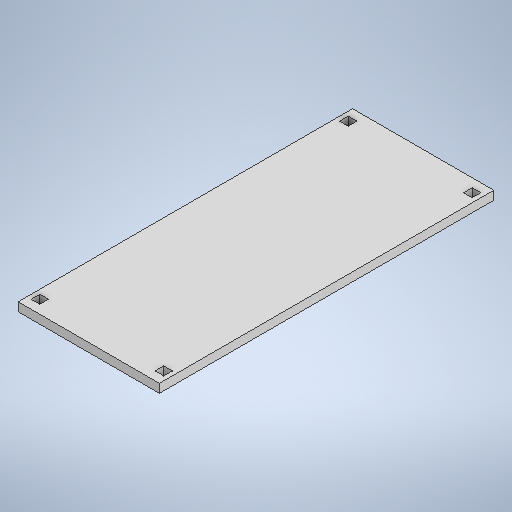
# Autodesk Inventor part: Platform_Arm_2
Saved by Autodesk Inventor 2025 (Build 290162000, 162)
## iProperties
Created: 2024-06-25
Part Number: Platform_Arm_2
Material: Generic
Document SubType Name: Modeling
Designer: User
Density: 1 g/cm^3
Appearance: Default
Author: User
Autodesk Inventor part; units mm, degrees
ref_plane "YZ Plane" through (0, 0, 0) normal (1, 0, 0) x (0, 1, 0)
ref_plane "XZ Plane" through (0, 0, 0) normal (0, 1, 0) x (-1, 0, 0)
ref_plane "XY Plane" through (0, 0, 0) normal (0, 0, 1) x (1, 0, 0)
sketch "Sketch1" plane through (0, 0, 0) normal (0, 1, 0) x (-1, 0, 0)
  line L0 (-245, 580) -> (245, 580)
  line L1 (245, 580) -> (245, -580)
  line L2 (245, -580) -> (-245, -580)
  line L3 (-245, -580) -> (-245, 580)
  line L4 (-245, 580) -> (245, -580) construction
  line L5 (245, 580) -> (-245, -580) construction
  line L6 (230, 550) -> (200, 550)
  line L7 (200, 550) -> (200, 520)
  line L8 (200, 520) -> (230, 520)
  line L9 (230, 520) -> (230, 550)
  line L10 (230, 550) -> (200, 520) construction
  line L11 (200, 550) -> (230, 520) construction
  line L12 (230, -520) -> (200, -520)
  line L13 (200, -520) -> (200, -550)
  line L14 (200, -550) -> (230, -550)
  line L15 (230, -550) -> (230, -520)
  line L16 (230, -520) -> (200, -550) construction
  line L17 (200, -520) -> (230, -550) construction
  line L18 (-200, 550) -> (-230, 550)
  line L19 (-230, 550) -> (-230, 520)
  line L20 (-230, 520) -> (-200, 520)
  line L21 (-200, 520) -> (-200, 550)
  line L22 (-200, 550) -> (-230, 520) construction
  line L23 (-230, 550) -> (-200, 520) construction
  line L24 (-230, -520) -> (-200, -520)
  line L25 (-200, -520) -> (-200, -550)
  line L26 (-200, -550) -> (-230, -550)
  line L27 (-230, -550) -> (-230, -520)
  line L28 (-230, -520) -> (-200, -550) construction
  line L29 (-200, -520) -> (-230, -550) construction
  point P0 (0, 0)
  point P1 (215, 535)
  point P2 (215, -535)
  point P3 (-215, 535)
  point P4 (230, 535)
  point P5 (215, 550)
  point P6 (-215, 550)
  point P7 (-230, 535)
  point P8 (215, -550)
  point P9 (230, -535)
  point P10 (-215, -535)
  dimension "d0" = 1160
  dimension "d1" = 490
  dimension "d2" = 30
  dimension "d3" = 30
  dimension "d4" = 15
  dimension "d5" = 30
  dimension "d6" = 30
  dimension "d7" = 15
  dimension "d8" = 30
  dimension "d9" = 15
  dimension "d10" = 30
  dimension "d11" = 30
  dimension "d12" = 15
  dimension "d13" = 30
  constraints: 60 end point, 16 midpoint, 10 parallel, 5 horizontal, 5 perpendicular, 4 equal length
  measures "d0" distance of L0.end L1.end
  measures "d1" distance of L1.end L2.end
  measures "d2" distance of L7.end L8.end
  measures "d3" distance of L8.end L6.start
  measures "d4" distance from line of L1 point (230, 535)
  measures "d5" distance from line of L0 point (215, 550)
  measures "d6" distance from line of L0 point (-215, 550)
  measures "d7" distance from line of L3 point (-230, 535)
  measures "d8" distance from line of L2 point (215, -550)
  measures "d9" distance from line of L1 point (230, -535)
  measures "d10" distance of L25.end L26.end
  measures "d11" distance of L24.end L25.end
  measures "d12" distance between parallel lines of L3 L27
  measures "d13" distance between parallel lines of L2 L26
extrude "Extrusion1" add sketch "Sketch1" along normal blind 30
sketch "Sketch2" plane through (0, 0, 0) normal (0, -1, 0) x (1, 0, 0)
  line L0 (-150, -325) -> (150, -325)
  line L1 (150, -325) -> (150, 325)
  line L2 (150, 325) -> (-150, 325)
  line L3 (-150, 325) -> (-150, -325)
  line L4 (-150, -325) -> (150, 325) construction
  line L5 (150, -325) -> (-150, 325) construction
  point P0 (0, 0)
  dimension "d16" = 650
  dimension "d17" = 300
  constraints: 12 end point, 2 midpoint, 2 parallel, 1 horizontal, 1 perpendicular
  measures "d16" distance of L0.end L1.end
  measures "d17" distance of L1.end L2.end
extrude "Extrusion2" add sketch "Sketch2" along normal blind 30
body "Solid1"
